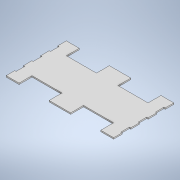
# Autodesk Inventor part: onderkant
Saved by Autodesk Inventor 2022 (Build 260153000, 153)
## iProperties
Created: 2021-12-16
Part Number: onderkant
Material: Generic
Document SubType Name: Modeling
Designer: keemi
Density: 1 g/cm^3
Appearance: Default
Author: keemi
Autodesk Inventor part; units mm, degrees
ref_plane "YZ Plane" through (0, 0, 0) normal (1, 0, 0) x (0, 1, 0)
ref_plane "XZ Plane" through (0, 0, 0) normal (0, 1, 0) x (-1, 0, 0)
ref_plane "XY Plane" through (0, 0, 0) normal (0, 0, 1) x (1, 0, 0)
sketch "Sketch1" plane through (0, 0, 0) normal (0, 1, 0) x (-1, 0, 0)
  line L0 (0, 0) -> (250, 0)
  line L1 (250, 0) -> (250, -140)
  line L2 (250, -140) -> (0, -140)
  line L3 (0, -140) -> (0, 0)
  dimension "d0" = 250
  dimension "d1" = 140
  constraints: 8 end point, 2 parallel, 1 horizontal, 1 perpendicular
  measures "d0" distance of L1.end L2.end
  measures "d1" distance of L0.end L1.end
extrude "Extrusion1" add sketch "Sketch1" along normal blind 3
sketch "Sketch8" plane through (0, 0, 0) normal (0, -1, 0) x (1, 0, 0)
  line L0 (0, -140) -> (-250, -140) projected
  line L1 (-250, -140) -> (-220, -140)
  line L2 (-220, -140) -> (-220, -110)
  line L3 (-220, -110) -> (-150, -110)
  line L4 (-220, -110) -> (-150, -110) construction
  line L5 (-150, -110) -> (-150, -140)
  line L6 (0, -140) -> (-30, -140)
  line L7 (0, -140) -> (-250, -140) projected
  line L8 (-30, -140) -> (-30, -110)
  line L9 (-30, -110) -> (-100, -110)
  line L10 (-100, -110) -> (-100, -140)
  line L11 (-250, -140) -> (-250, -70)
  line L12 (-250, -70) -> (24.9367, -70)
  line L13 (-97, 0) -> (-250, 0)
  line L14 (-250, 0) -> (-220, 0)
  line L15 (-220, 0) -> (-220, -30)
  line L16 (-220, -30) -> (-150, -30)
  line L17 (-220, -30) -> (-150, -30) construction
  line L18 (-150, -30) -> (-150, 0)
  line L19 (0, 0) -> (-30, 0)
  line L20 (0, 0) -> (-27, 0)
  line L21 (-30, 0) -> (-30, -30)
  line L22 (-30, -30) -> (-100, -30)
  line L23 (-100, -30) -> (-100, 0)
  line L24 (0, -140) -> (-250, -140)
  point P0 (-97, -140)
  point P1 (-27, -140)
  dimension "d64" = 30
  dimension "d65" = 30
  dimension "d66" = 70
  dimension "d67" = 0
  dimension "d68" = 30
  dimension "d69" = 30
  dimension "d70" = 70
  dimension "d71" = 70
  constraints: 47 end point, 14 symmetric about line, 11 point on line, 4 perpendicular, 2 collinear, 2 horizontal, 1 vertical
  measures "d64" distance of L0.end L1.end
  measures "d65" distance of L1.end L2.end
  measures "d66" distance of L2.end L3.end
  measures "d67" distance between parallel lines of L3 L4
  measures "d68" distance of L0.start L6.end
  measures "d69" distance of L6.end L8.end
  measures "d70" distance of L8.end L9.end
  measures "d71" distance of L0.end L11.end
extrude "Extrusion7" cut sketch "Sketch8" against normal blind 10
sketch "Sketch9" plane through (0, 0, 0) normal (0, -1, 0) x (1, 0, 0)
  line L0 (0, 0) -> (-30, 0)
  line L1 (-30, 0) -> (-30, -30)
  line L2 (-30, -30) -> (-100, -30)
  line L3 (-100, -30) -> (-100, 0)
  line L4 (-30, 0) -> (-100, 0)
  line L5 (-150, 0) -> (0, 0) projected
  dimension "d74" = 30
  dimension "d75" = 30
  dimension "d76" = 70
  constraints: 10 end point, 3 perpendicular, 1 collinear, 1 horizontal, 1 point on line
  measures "d74" distance of L0.start L0.end
  measures "d75" distance of L0.end L1.end
  measures "d76" distance of L1.end L2.end
extrude "Extrusion8" cut sketch "Sketch9" against normal blind 10
sketch "Sketch10" plane through (0, 0, 0) normal (0, -1, 0) x (1, 0, 0)
  line L0 (0, 0) -> (0, -20)
  line L1 (0, 0) -> (0, -140) projected
  line L2 (0, -20) -> (-3, -20)
  line L3 (-3, -20) -> (-3, -40)
  line L4 (-3, -40) -> (0, -40)
  line L5 (0, -40) -> (0, -60)
  line L6 (0, -60) -> (-3, -60)
  line L7 (-3, -60) -> (-3, -80)
  line L8 (-3, -80) -> (0, -80)
  line L9 (0, -80) -> (0, -100)
  line L10 (0, -100) -> (-3, -100)
  line L11 (-3, -100) -> (-3, -120)
  line L12 (-3, -120) -> (0, -120)
  line L13 (0, 0) -> (-125, 0)
  line L14 (-250, -140) -> (-250, 0) projected
  line L15 (-125, 0) -> (-125, -140)
  line L16 (-250, -20) -> (-247, -20)
  line L17 (-247, -20) -> (-247, -40)
  line L18 (-247, -40) -> (-250, -40)
  line L19 (-250, -40) -> (-250, -60)
  line L20 (-250, -60) -> (-247, -60)
  line L21 (-247, -60) -> (-247, -80)
  line L22 (-247, -80) -> (-250, -80)
  line L23 (-250, -80) -> (-250, -100)
  line L24 (-250, -100) -> (-247, -100)
  line L25 (-247, -100) -> (-247, -120)
  line L26 (-247, -120) -> (-250, -120)
  dimension "d79" = 20
  dimension "d80" = 3
  dimension "d81" = 20
  dimension "d82" = 20
  dimension "d83" = 3
  dimension "d84" = 20
  dimension "d85" = 20
  dimension "d86" = 20
  dimension "d87" = 125
  constraints: 50 end point, 16 point on line, 12 symmetric about line, 8 perpendicular
  measures "d79" distance of L0.start L0.end
  measures "d80" distance of L0.end L2.end
  measures "d81" distance of L2.end L3.end
  measures "d82" distance of L4.end L5.end
  measures "d83" distance of L5.end L6.end
  measures "d84" distance of L6.end L7.end
  measures "d85" distance of L8.end L9.end
  measures "d86" distance of L10.end L11.end
  measures "d87" distance of L0.start L13.end
extrude "Extrusion9" cut sketch "Sketch10" against normal blind 10
body "Solid1"
